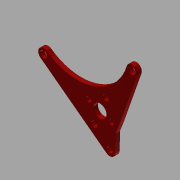
# Autodesk Inventor part: OutlineSketch1
Saved by Autodesk Inventor 2013 (Build 170138000, 138)
## iProperties
Created: 2013-06-03
Part Number: OutlineSketch1
Material: Aluminum 6061
Document SubType Name: Modeling
Designer: mvarma
Density: 2.71 g/cm^3
Author: mvarma
Autodesk Inventor part; units mm, degrees
ref_plane "YZ Plane" through (0, 0, 0) normal (1, 0, 0) x (0, 1, 0)
ref_plane "XZ Plane" through (0, 0, 0) normal (0, 1, 0) x (-1, 0, 0)
ref_plane "XY Plane" through (0, 0, 0) normal (0, 0, 1) x (1, 0, 0)
sketch "Sketch1" plane through (0, 0, 0) normal (0, 0, 1) x (1, 0, 0)
  line L0 (0, 0) -> (304.8, 0) construction
  line L1 (304.8, 0) -> (304.8, 50.8) construction
  line L2 (304.8, 50.8) -> (0, 50.8) construction
  line L3 (0, 50.8) -> (0, 0) construction
  circle A0 centre (152.4, 23.8125) radius 6.35 construction
  circle A1 centre (152.4, 23.8125) radius 34.29 construction
  circle A2 centre (152.4, 23.8125) radius 22.225 construction
  line L4 (152.4, 23.8125) -> (139.8147, 61.8398) construction
  circle A3 centre (139.8147, 61.8398) radius 9.525 construction
  circle A4 centre (139.8147, 61.8398) radius 17.78 construction
  circle A5 centre (91.4913, 85.598) radius 32.258 construction
  circle A6 centre (164.4242, 109.7354) radius 32.258 construction
  line L5 (0, 50.8) -> (0, 53.34) construction
  line L6 (0, 53.34) -> (304.8, 53.34) construction
  line L7 (304.8, 53.34) -> (304.8, 50.8) construction
  circle A7 centre (139.8147, 61.8398) radius 21.59 construction
  circle A8 centre (152.4, 23.8125) radius 46.99 construction
  circle A9 centre (152.4, 23.8125) radius 50.8 construction
  arc A10 (86.31, 79.9698) -> (92.3737, 93.1969) centre (91.4913, 85.598) ccw construction
  circle A11 centre (164.4242, 109.7354) radius 7.65 construction
  circle A12 centre (164.4242, 109.7354) radius 9.1 construction
  circle A13 centre (139.8147, 61.8398) radius 22.9 construction
  line L8 (86.31, 79.9698) -> (124.3047, 44.992) construction
  line L9 (171.9401, 108.3093) -> (162.3134, 57.5711) construction
  line L10 (92.3737, 93.1969) -> (91.4913, 85.598) construction
  line L11 (91.4913, 85.598) -> (86.31, 79.9698) construction
  arc A14 (129.415, 93.2634) -> (131.9683, 98.1756) centre (128.1681, 97.0312) ccw
  circle A15 centre (128.1681, 97.0312) radius 7.9375 construction
  line L12 (92.3737, 93.1969) -> (127.2525, 89.1467) construction
  line L13 (133.6065, 91.2495) -> (159.1828, 115.3076) construction
  line L14 (159.1828, 115.3076) -> (164.4242, 109.7354) construction
  line L15 (171.9401, 108.3093) -> (164.4242, 109.7354) construction
  line L16 (139.8147, 61.8398) -> (128.1681, 97.0312) construction
  line L17 (91.4913, 85.598) -> (164.4242, 109.7354) construction
  line L18 (152.4, 23.8125) -> (91.4913, 85.598) construction
  line L19 (152.4, 23.8125) -> (164.4242, 109.7354) construction
  circle A16 centre (128.1681, 97.0312) radius 9.2075 construction
  circle A17 centre (128.1681, 97.0312) radius 6.1595 construction
  arc A18 (92.3737, 93.1969) -> (86.31, 79.9698) centre (91.4913, 85.598) ccw construction
  circle A19 centre (164.4242, 109.7354) radius 25.4 construction
  line L20 (104.9341, 114.9215) -> (78.0485, 56.2745) construction
  circle A20 centre (91.4913, 85.598) radius 25.4 construction
  line L21 (104.3539, 107.5736) -> (92.6302, 85.0411) construction
  line L22 (80.9064, 62.5086) -> (90.326, 86.0974) construction
  arc A21 (100.6288, 111.8976) -> (98.8626, 107.4747) centre (99.7457, 109.6862) ccw construction
  arc A22 (103.2548, 105.4612) -> (105.453, 109.686) centre (104.3539, 107.5736) ccw construction
  arc A23 (103.2548, 105.4612) -> (98.8626, 107.4747) centre (80.9064, 62.5086) ccw construction
  line L23 (99.7457, 109.6862) -> (100.6288, 111.8976) construction
  line L24 (104.3539, 107.5736) -> (105.453, 109.686) construction
  arc A24 (105.453, 109.686) -> (100.6288, 111.8976) centre (80.9064, 62.5086) ccw construction
  arc A25 (87.9407, 76.0281) -> (97.3197, 94.0541) centre (92.6302, 85.0411) ccw construction
  line L25 (90.326, 86.0974) -> (99.7457, 109.6862) construction
  line L26 (92.6302, 85.0411) -> (80.9064, 62.5086) construction
  arc A26 (87.9407, 76.0281) -> (86.5582, 76.6619) centre (80.9064, 62.5086) ccw construction
  arc A27 (97.3197, 94.0541) -> (94.0939, 95.5329) centre (80.9064, 62.5086) ccw construction
  arc A28 (94.0939, 95.5329) -> (86.5582, 76.6619) centre (90.326, 86.0974) ccw construction
  line L27 (164.4242, 109.7354) -> (142.1549, 121.9516) construction
  line L28 (164.4242, 109.7354) -> (186.6936, 97.5192) construction
  circle A29 centre (139.8147, 61.8398) radius 26.71 construction
  circle A30 centre (152.4, 23.8125) radius 11.176 construction
  line L29 (152.4, 23.8125) -> (159.3829, 2.713) construction
  circle A31 centre (152.4, 23.8125) radius 4.7625
  line L30 (156.5446, 34.1916) -> (148.2554, 13.4334) construction
  circle A32 centre (156.5446, 34.1916) radius 2.1082
  circle A33 centre (148.2554, 13.4334) radius 2.1082
  arc A34 (166.3853, 21.8496) -> (163.8906, 15.6022) centre (152.4, 23.8125) ccw
  circle A35 centre (111.4232, 39.3255) radius 9.525 construction
  circle A36 centre (176.0321, 60.708) radius 9.525 construction
  arc A37 (113.755, 42.537) -> (109.015, 36.1709) centre (111.4232, 39.3255) ccw
  arc A38 (179.7701, 59.3747) -> (172.2448, 61.8944) centre (176.0321, 60.708) ccw
  arc A39 (158.136, 6.4808) -> (156.9747, -0.4416) centre (159.3829, 2.713) ccw
  line L31 (152.4, 23.8125) -> (165.1379, 18.7259) construction
  line L32 (166.3853, 21.8496) -> (163.8906, 15.6022)
  arc A40 (163.8906, 15.6022) -> (166.3853, 21.8496) centre (152.4, 23.8125) ccw construction
  line L33 (163.8906, 15.6022) -> (163.3483, 2.5483)
  line L34 (156.9747, -0.4416) -> (109.015, 36.1709)
  line L35 (166.3853, 21.8496) -> (179.7701, 59.3747)
  arc A41 (124.3867, 95.8262) -> (129.415, 93.2634) centre (128.1681, 97.0312) ccw
  arc A42 (131.9683, 98.1756) -> (124.3867, 95.8262) centre (128.1681, 97.0312) ccw
  arc A43 (131.7101, 98.9085) -> (131.9683, 98.1756) centre (178.947, 115.132) ccw
  arc A44 (163.3483, 2.5483) -> (158.136, 6.4808) centre (159.3829, 2.713) ccw
  arc A45 (156.9747, -0.4416) -> (163.3483, 2.5483) centre (159.3829, 2.713) ccw
  circle A46 centre (136.0438, 73.2342) radius 37.9355
  point P0 (102.0762, 108.6874)
  point P1 (145.0256, 46.8513)
  dimension "d1" = 50.8
  dimension "d3" = 23.8125
  dimension "d4" = 152.4
  dimension "d7" = 68.58
  dimension "d8" = 44.45
  dimension "d9" = 19.05
  dimension "d10" = 35.56
  dimension "d11" = 40.0558
  dimension "d12" = 64.516
  dimension "d13" = 64.516
  dimension "d15" = 2.54
  dimension "d16" = 304.8
  dimension "d17" = 43.18
  dimension "d18" = 93.98
  dimension "d19" = 101.6
  dimension "d21" = 15.3
  dimension "d22" = 15.3
  dimension "d24" = 18.2
  dimension "d29" = 45.8
  dimension "d30" = 143.991
  dimension "d31" = 7.9375
  dimension "d32" = 15.875
  dimension "d33" = 143.991
  dimension "d35" = 18.415
  dimension "d37" = 12.319
  dimension "d40" = 50.8
  dimension "d42" = 18.004
  dimension "d43" = 18.004
  dimension "d44" = 50.8
  dimension "d75" = 2.86
  dimension "d80" = 4.7625
  dimension "d82" = 4.7625
  dimension "d83" = 50.8
  dimension "d84" = 50.8
  dimension "d97" = 48.4188
  dimension "d99" = 20.32
  dimension "d101" = 25.4
  dimension "d102" = 25.4
  dimension "d103" = 10.16
  dimension "d105" = 18.004
  dimension "d106" = 18.004
  dimension "d107" = 53.42
  dimension "d149" = 22.352
  dimension "d152" = 180
  dimension "d163" = 9.525
  dimension "d190" = 12.7
  dimension "d191" = 4.2164
  dimension "d192" = 4.2164
  dimension "d209" = 28.2448
  dimension "d210" = 19.05
  dimension "d211" = 19.05
  dimension "d212" = 7.9375
  dimension "d214" = 22.225
  dimension "d215" = 7.9375
  dimension "d216" = 13.716
  dimension "d232" = 3.9688
  constraints: 74 end point, 59 point on circle, 47 centre point, 31 coincident, 24 tangent, 10 point on line, 7 collinear, 7 perpendicular, 4 parallel, 3 midpoint, 1 horizontal, 1 symmetric about line, 2 other
  measures "d1" distance of L1.end L0.end
  measures "d3" distance from line of L0 A0.centre
  measures "d4" distance from line of L3 A0.centre
  measures "d7" diameter of A1
  measures "d8" diameter of A2
  measures "d9" diameter of A3
  measures "d10" diameter of A4
  measures "d11" distance of L4.start L4.end
  measures "d12" diameter of A5
  measures "d13" diameter of A6
  measures "d15" distance of L2.end L5.end
  measures "d16" distance of L0.end L0.start
  measures "d17" diameter of A7
  measures "d18" diameter of A8
  measures "d19" diameter of A9
  measures "d21" diameter of A10
  measures "d22" diameter of A11
  measures "d24" diameter of A12
  measures "d29" diameter of A13
  measures "d30" angle of L11 L10
  measures "d31" diameter of A14
  measures "d32" diameter of A15
  measures "d33" angle of L15 L14
  measures "d35" diameter of A16
  measures "d37" diameter of A17
  measures "d40" diameter of A19
  measures "d42" angle of L10 L20
  measures "d43" angle of L11 L20
  measures "d44" diameter of A20
  measures "d75" angle of L20 L21
  measures "d80" diameter of A21
  measures "d82" diameter of A22
  measures "d83" distance of L22.start L25.end
  measures "d84" distance of L21.start L22.start
  measures "d97" radius of A23
  measures "d99" diameter of A25
  measures "d101" distance of L22.start L22.end
  measures "d102" distance of L21.end L22.start
  measures "d103" radius of A28
  measures "d105" angle of L27 L14
  measures "d106" angle of L28 L15
  measures "d107" diameter of A29
  measures "d149" diameter of A30
  measures "d152" angle of L29 L4
  measures "d163" diameter of A31
  measures "d190" diameter of A0
  measures "d191" diameter of A32
  measures "d192" diameter of A33
  measures "d209" diameter of A34
  measures "d210" diameter of A35
  measures "d211" diameter of A36
  measures "d212" diameter of A37
  measures "d214" distance of A0.centre L29.end
  measures "d215" diameter of A39
  measures "d216" distance of L31.start L31.end
  measures "d232" radius of A38
extrude "Extrusion3" add sketch "Sketch1" along normal blind 3.175 contours L32 A34 | A34 A46 A38 L35 | A34 L33 A44 A39 L34 A37 A46 | A45 A39 A44
hole "Hole3" at (80.9064, 62.5086, 0) at (186.6936, 97.5192, 0) at (128.1681, 97.0312, 0) at (111.4232, 39.3255, 0) at (176.0321, 60.708, 0) direction (0, 0, 1) diameter 4.9784 end through all clearance for "Socket Head Cap Screw" size "#10" standard "Ansi Unified Screw Threads"
fillet "Fillet3" radius 3.175 2 edges at (166.3853, 21.8496, 1.5875) (163.8906, 15.6022, 1.5875)
hole "Hole6" at (159.3829, 2.713, 0) direction (0, 0, 1) diameter 4.318 end through all clearance for "Socket Head Cap Screw" size "#8" standard "Ansi Unified Screw Threads"
sketch "Sketch5" plane through (0, 0, 3.175) normal (0, 0, 1) x (1, 0, 0)
  line L0 (164.0917, 16.1059) -> (166.3634, 21.7946) projected
  circle A0 centre (156.5446, 34.1916) radius 2.1082 projected
  circle A1 centre (148.2554, 13.4334) radius 2.1082 projected
  circle A2 centre (152.4, 23.8125) radius 4.7625 projected
  circle A3 centre (152.4, 23.8125) radius 8.7313 construction
  line L1 (156.5446, 34.1916) -> (148.2554, 13.4334) construction
  line L2 (144.2914, 27.0505) -> (160.5086, 20.5745) construction
  point P0 (0, 0)
  point P1 (152.4, 23.8125)
  dimension "d240" = 17.4625
  constraints: 4 end point, 3 coincident, 2 midpoint, 2 point on circle, 1 centre point, 1 parallel, 1 perpendicular
  measures "d240" diameter of A3
hole "Hole7" at (144.2914, 27.0505, 3.175) at (160.5086, 20.5745, 3.175) direction (0, 0, -1) diameter 3.5719 end through all
equation "\"d8\" = Gear35tPD"
equation "\"d9\" = Gear15tPD"
equation "\"d10\" = Gear28tPD"
equation "\"d11\" = 0.5 * Gear48tPD + 0.5 * Gear15tPD + MeshingClearance"
equation "\"d12\" = CimOD"
equation "\"d13\" = CimOD"
equation "\"d17\" = Gear28tPD + ClearanceDiameter"
equation "\"d18\" = WheelOD"
equation "\"d19\" = WheelClearance"
equation "\"Pulley48tPD\" = 45.8"
equation "\"Pulley19tPD\" = 18.2"
equation "\"Pulley16tPD\" = 15.3"
equation "\"Gear15tPD\" = 19.05"
equation "\"Gear35tPD\" = 44.45"
equation "\"Gear48tPD\" = 60.96"
equation "\"Gear28tPD\" = 35.56"
equation "\"BearingLargeOD\" = 28.575"
equation "\"BearingSmallOD\" = 22.225"
equation "\"MeshingClearance\" = 0.0508"
equation "\"CimOD\" = 64.516"
equation "\"WheelOD\" = 93.98"
equation "\"ClearanceDiameter\" = 7.62"
equation "\"WheelClearance\" = 101.6"
equation "\"TensioningBearingID\" = 6.35"
equation "\"TensioningBearingOD\" = 15.875"
equation "\"SpingClipClearance\" = 8.89"
equation "\"Pi\" = 79.79645"
equation "\"Pulley56tPD\" = 53.5"
equation "\"BearingXLargeOD\" = 34.925"
body "Solid3"
